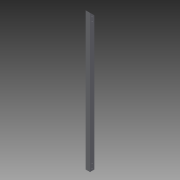
# Autodesk Inventor part: 1x1 support
Saved by Autodesk Inventor 2015 SP1 (Build 190203100, 203)
## iProperties
Created: 2015-01-17
Part Number: 1x1 support
Material: Generic
Document SubType Name: Modeling
Designer: Jarod
Density: 1 g/cm^3
Appearance: Default
Author: Jarod
Autodesk Inventor part; units mm, degrees
ref_plane "YZ Plane" through (0, 0, 0) normal (1, 0, 0) x (0, 1, 0)
ref_plane "XZ Plane" through (0, 0, 0) normal (0, 1, 0) x (-1, 0, 0)
ref_plane "XY Plane" through (0, 0, 0) normal (0, 0, 1) x (1, 0, 0)
sketch "Sketch1" plane through (0, 0, 0) normal (0, 1, 0) x (-1, 0, 0)
  line L0 (0, 0) -> (25.4, 0)
  line L1 (25.4, 0) -> (25.4, -25.4)
  line L2 (25.4, -25.4) -> (0, -25.4)
  line L3 (0, -25.4) -> (0, 0)
  line L4 (3.175, -3.175) -> (22.225, -3.175)
  line L5 (22.225, -3.175) -> (22.225, -22.225)
  line L6 (22.225, -22.225) -> (3.175, -22.225)
  line L7 (3.175, -22.225) -> (3.175, -3.175)
  dimension "d0" = 25.4
  dimension "d1" = 25.4
  dimension "d2" = 19.05
  dimension "d3" = 19.05
  dimension "d4" = 3.175
  dimension "d5" = 3.175
  constraints: 16 end point, 4 parallel, 2 horizontal, 2 perpendicular
  measures "d0" distance of L1.end L2.end
  measures "d1" distance of L0.end L1.end
  measures "d2" distance of L5.end L6.end
  measures "d3" distance of L4.end L5.end
  measures "d4" distance between parallel lines of L3 L7
  measures "d5" distance between parallel lines of L0 L4
extrude "Extrusion1" add sketch "Sketch1" along normal blind 850.9
sketch "Sketch2" plane through (-25.4, 0, -25.4) normal (-1, 0, 0) x (0, 0, 1)
  line L0 (25.4, 0) -> (0, 0) projected
  line L1 (25.4, 0) -> (25.4, 850.9) projected
  line L2 (0, 850.9) -> (25.4, 850.9) projected
  line L3 (0, 0) -> (0, 850.9) projected
  point P0 (12.7, 812.8)
  point P1 (12.7, 787.4)
  point P2 (12.7, 12.7)
  point P3 (12.7, 38.1)
  dimension "d8" = 12.7
  dimension "d9" = 38.1
  dimension "d12" = 12.7
  dimension "d13" = 12.7
  dimension "d14" = 12.7
  dimension "d15" = 12.7
  dimension "d23" = 812.8
  dimension "d24" = 787.4
  measures "d8" distance from line of L0 point (12.7, 12.7)
  measures "d9" distance from line of point (12.7, 38.1) L0
  measures "d12" distance from line of L3 point (12.7, 787.4)
  measures "d13" distance from line of L3 point (12.7, 812.8)
  measures "d14" distance from line of L3 point (12.7, 12.7)
  measures "d15" distance from line of L3 point (12.7, 38.1)
  measures "d23" distance from line of L0 point (12.7, 812.8)
  measures "d24" distance from line of L0 point (12.7, 787.4)
hole "Hole1" at (-25.4, 812.8, -12.7) at (-25.4, 787.4, -12.7) at (-25.4, 12.7, -12.7) at (-25.4, 38.1, -12.7) direction (1, 0, 0) diameter 3.9688 end through all
sketch "Sketch3" plane through (-25.4, 0, -25.4) normal (-1, 0, 0) x (0, 0, 1)
  circle A0 centre (12.7, 12.7) radius 1.9844 projected
  circle A1 centre (12.7, 812.8) radius 1.9844 projected
  circle A2 centre (12.7, 787.4) radius 1.9844 projected
  circle A3 centre (12.7, 38.1) radius 1.9844 projected
  line L0 (25.4, 0) -> (0, 0) projected
  line L1 (25.4, 0) -> (25.4, 850.9) projected
  line L2 (0, 850.9) -> (25.4, 850.9) projected
  line L3 (0, 0) -> (0, 850.9) projected
  line L4 (25.4, 850.9) -> (0, 850.9)
  line L5 (0, 850.9) -> (0, 812.8)
  line L6 (0, 0) -> (0, 850.9) projected
  line L7 (0, 812.8) -> (25.4, 850.9)
  dimension "d25" = 38.1
  constraints: 6 end point, 1 horizontal, 1 point on line
  measures "d25" distance of L2.start L5.end
extrude "Extrusion2" cut sketch "Sketch3" against normal blind 25.4 contours L7 L3 L2
body "Solid1"
